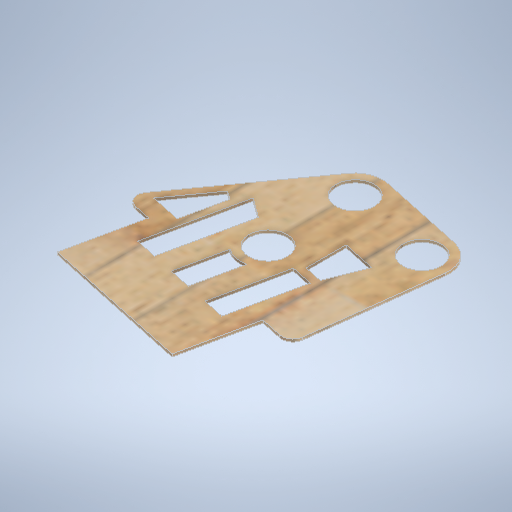
# Autodesk Inventor part: gear_plate_base
Saved by Autodesk Inventor 2026.1 (Build 301233020, 233B)
## iProperties
Created: 2024-04-01
Part Number: gear_plate_base
Material: 木材 (カエデ材)
Document SubType Name: Modeling
Designer: hibik
Density: 0.67 g/cm^3
Appearance: ナチュラル カエデ材 - 光沢 濃い着色
Author: hibik
Autodesk Inventor part; units mm, degrees
ref_plane "YZ Plane" through (0, 0, 0) normal (1, 0, 0) x (0, 1, 0)
ref_plane "XZ Plane" through (0, 0, 0) normal (0, 1, 0) x (-1, 0, 0)
ref_plane "XY Plane" through (0, 0, 0) normal (0, 0, 1) x (1, 0, 0)
sketch "スケッチ1" plane through (0, 0, 0) normal (0, 1, 0) x (-1, 0, 0)
  line L0 (25, 0) -> (-25, 0)
  line L1 (-25, 0) -> (-25, -104.5)
  line L2 (-25, -104.5) -> (25, -104.5) construction
  line L3 (25, -104.5) -> (25, 0)
  circle A0 centre (0, 0) radius 25
  circle A1 centre (0, 0) radius 57 construction
  circle A2 centre (0, -79.5) radius 22.5 construction
  circle A3 centre (0, 0) radius 75 construction
  circle A4 centre (0, -79.5) radius 10.75
  circle A5 centre (0, 0) radius 10.75
  circle A6 centre (-77.7461, -62.8931) radius 25
  circle A7 centre (-77.7461, -62.8931) radius 10.75
  circle A8 centre (0, -79.5) radius 25
  line L4 (-5.2223, -103.9485) -> (-82.9684, -87.3415)
  line L5 (-72.5238, -38.4446) -> (5.2223, -55.0515)
  line L6 (-77.7461, -62.8931) -> (-82.9684, -87.3415)
  point P0 (25, -79.5)
  point P1 (-25, -48.5959)
  dimension "d0" = 114
  dimension "d1" = 45
  dimension "d2" = 150
  dimension "d4" = 21.5
  dimension "d5" = 50
  dimension "d25" = 79.5
  constraints: 14 end point, 9 centre point, 9 tangent, 8 coincident, 5 point on circle, 3 equal radius, 2 parallel, 2 perpendicular, 1 horizontal, 1 midpoint, 1 vertical alignment
  measures "d0" diameter of A1
  measures "d1" diameter of A2
  measures "d2" diameter of A3
  measures "d4" diameter of A5
  measures "d5" distance of L1.end L2.end
  measures "d25" distance from line of A2.centre L6
extrude "押し出し1" add sketch "スケッチ1" along normal blind 2.5 contours A0 L0 A5 | L0 A5 A0 | L3 A8 L5 L1 A0 | A8 | A8 L1 L5 | L4 L1 A8 | L1 L4 A6 L5 | A6
sketch "スケッチ4" plane through (0, 2.5, 0) normal (0, 1, 0) x (1, 0, 0)
  line L0 (-1, 90.2034) -> (1, 90.2034)
  line L1 (1, 90.2034) -> (1, 96.5)
  line L2 (1, 96.5) -> (-1, 96.5)
  line L3 (-1, 96.5) -> (-1, 90.2034)
  arc A0 (-25, 0) -> (25, 0) centre (0, 0) ccw projected
  line L4 (25, 0) -> (25, 48.5959) projected
  line L5 (25, 48.5959) -> (72.5238, 38.4446) projected
  arc A1 (72.5238, 38.4446) -> (82.9684, 87.3415) centre (77.7461, 62.8931) ccw projected
  line L6 (82.9684, 87.3415) -> (5.2223, 103.9485) projected
  arc A2 (5.2223, 103.9485) -> (-25, 79.5) centre (0, 79.5) ccw projected
  line L7 (-25, 79.5) -> (-25, 0) projected
  circle A3 centre (0, 0) radius 10.75 projected
  circle A4 centre (77.7461, 62.8931) radius 10.75 projected
  circle A5 centre (0, 79.5) radius 10.75 projected
  circle A6 centre (0, 79.5) radius 10.75 projected
  line L8 (-16.9706, -1) -> (16.9706, -1)
  line L9 (16.9706, -1) -> (16.9706, 1)
  line L10 (16.9706, 1) -> (-16.9706, 1)
  line L11 (-16.9706, 1) -> (-16.9706, -1)
  line L12 (-1, -16.9706) -> (1, -16.9706)
  line L13 (1, -16.9706) -> (1, 16.9706)
  line L14 (1, 16.9706) -> (-1, 16.9706)
  line L15 (-1, 16.9706) -> (-1, -16.9706)
  circle A7 centre (0, 0) radius 17
  point P0 (0, 96.5)
  point P1 (-16.9706, 0)
  point P2 (0, 16.9706)
  point P3 (-1, -10.7034)
  point P4 (1, -10.7034)
  point P5 (10.7034, 1)
  point P6 (10.7034, -1)
  point P7 (-1, 10.7034)
  point P8 (1, 10.7034)
  point P9 (-10.7034, -1)
  point P10 (-10.7034, 1)
  dimension "d26" = 17
  dimension "d27" = 2
  dimension "d30" = 34
  constraints: 24 end point, 6 parallel, 5 perpendicular, 4 point on circle, 3 horizontal, 3 midpoint, 2 vertical alignment, 1 centre point, 1 coincident, 1 horizontal alignment, 2 other
  measures "d26" distance from line of L2 A2.centre
  measures "d27" distance of L1.end L2.end
  measures "d30" diameter of A7
extrude "押し出し4" cut sketch "スケッチ4" against normal through all contours A5 L0 | L3 L2 L1 A5 | A3 L10 L9 L8 | A3 L15 L14 L13 | L13 L12 L15 A3 | A3 L8 L11 L10 picked at (-0.1113, 90.2172)
sketch "スケッチ5" plane through (0, 2.5, 0) normal (0, 1, 0) x (1, 0, 0)
  circle A0 centre (0, 0) radius 17.5
  circle A1 centre (0, 79.5) radius 17.5
  circle A2 centre (77.7461, 62.8931) radius 17.5
  arc A3 (-1, 90.2034) -> (1, 90.2034) centre (0, 79.5) ccw projected
  circle A4 centre (77.7461, 62.8931) radius 10.75 projected
  dimension "d31" = 35
  dimension "d32" = 35
  dimension "d33" = 35
  constraints: 3 centre point, 2 concentric, 1 coincident
  measures "d31" diameter of A0
  measures "d32" diameter of A1
  measures "d33" diameter of A2
extrude "押し出し5" cut sketch "スケッチ5" against normal through all contours A0 | A1 | A2 | A4
sketch "スケッチ7" plane through (0, 2.5, 0) normal (0, 1, 0) x (1, 0, 0)
  line L0 (62.2228, 90.7503) -> (63.2008, 90.5415) projected
  line L1 (62.7118, 90.6459) -> (67.0985, 111.1826)
  line L2 (9.4001, 123.5072) -> (87.1463, 106.9003) projected
  circle A0 centre (50.445, 105.0256) radius 1.75
  circle A1 centre (21.1068, 111.2923) radius 1.75
  point P0 (0, 0)
  dimension "d39" = 9.5
  dimension "d40" = 3.5
  dimension "d41" = 15
  dimension "d42" = 45
  dimension "d43" = 9.5
  constraints: 2 centre point, 2 end point, 1 equal radius, 1 midpoint, 1 perpendicular, 1 point on line
  measures "d39" distance from line of A0.centre L2
  measures "d40" diameter of A0
  measures "d41" distance from line of L1 A0.centre
  measures "d42" distance from line of A1.centre L1
  measures "d43" distance from line of L2 A1.centre
extrude "押し出し7" cut sketch "スケッチ7" against normal through all
sketch "スケッチ8" plane through (0, 2.5, 0) normal (0, 1, 0) x (1, 0, 0)
  line L0 (15.7233, -19.4365) -> (93.4694, 43.4566)
  arc A0 (-25, 0) -> (25, 0) centre (0, 0) ccw projected
  arc A1 (72.5238, 38.4446) -> (82.9684, 87.3415) centre (77.7461, 62.8931) ccw projected
  line L1 (25, 0) -> (25, 42.4151) projected
  line L2 (25, 0) -> (25, 48.5959) projected
  line L3 (25, 48.5959) -> (72.5238, 38.4446) projected
  constraints: 2 end point, 2 point on circle, 2 tangent
extrude "押し出し8" add sketch "スケッチ8" against normal up to surface (2.5 mm away)
sketch "スケッチ11" plane through (0, 2.5, 0) normal (0, 1, 0) x (1, 0, 0)
  line L0 (57.451, -61.3546) -> (47.0063, -110.2515) projected
  line L1 (86.7891, -67.6214) -> (57.451, -61.3546) projected
  line L2 (57.5442, -204.5328) -> (86.7891, -67.6214) projected
  line L3 (42.8751, -201.3994) -> (57.5442, -204.5328) projected
  line L4 (58.542, -128.054) -> (42.8751, -201.3994) projected
  arc A0 (58.542, -128.054) -> (47.0063, -110.2515) centre (43.873, -124.9206) ccw projected
  arc A1 (-87.9492, -81.4244) -> (-105.7517, -92.9601) centre (-91.0826, -96.0935) ccw projected
  line L5 (-105.7517, -92.9601) -> (-121.4186, -166.3055) projected
  line L6 (-121.4186, -166.3055) -> (-136.0876, -163.1722) projected
  line L7 (-136.0876, -163.1722) -> (-106.8428, -26.2607) projected
  line L8 (-106.8428, -26.2607) -> (-77.5046, -32.5275) projected
  line L9 (-77.5046, -32.5275) -> (-87.9492, -81.4244) projected
  line L10 (-117.2874, -75.1577) -> (76.3445, -116.5183) projected
  line L11 (-111.0206, -45.8195) -> (-117.2874, -75.1577) projected
  line L12 (-81.6824, -52.0863) -> (-111.0206, -45.8195) projected
  line L13 (-84.8158, -66.7554) -> (-81.6824, -52.0863) projected
  line L14 (50.1397, -95.5825) -> (-84.8158, -66.7554) projected
  line L15 (53.2731, -80.9134) -> (50.1397, -95.5825) projected
  line L16 (82.6113, -87.1801) -> (53.2731, -80.9134) projected
  line L17 (76.3445, -116.5183) -> (82.6113, -87.1801) projected
  line L18 (-99.6213, -36.495) -> (-103.0441, -35.7639) projected
  line L19 (-103.0441, -35.7639) -> (-103.6708, -38.6977) projected
  line L20 (-103.6708, -38.6977) -> (-100.248, -39.4288) projected
  line L21 (-100.248, -39.4288) -> (-100.9791, -42.8516) projected
  line L22 (-100.9791, -42.8516) -> (-98.0453, -43.4783) projected
  line L23 (-98.0453, -43.4783) -> (-97.3142, -40.0555) projected
  line L24 (-97.3142, -40.0555) -> (-93.8914, -40.7866) projected
  line L25 (-93.8914, -40.7866) -> (-93.2647, -37.8528) projected
  line L26 (-93.2647, -37.8528) -> (-96.6875, -37.1217) projected
  line L27 (-96.6875, -37.1217) -> (-95.9564, -33.6989) projected
  line L28 (-95.9564, -33.6989) -> (-98.8902, -33.0722) projected
  line L29 (-98.8902, -33.0722) -> (-99.6213, -36.495) projected
  line L30 (69.0332, -75.5881) -> (72.456, -76.3192) projected
  line L31 (72.456, -76.3192) -> (71.7249, -79.742) projected
  line L32 (71.7249, -79.742) -> (74.6587, -80.3686) projected
  line L33 (74.6587, -80.3686) -> (75.3898, -76.9459) projected
  line L34 (75.3898, -76.9459) -> (78.8126, -77.677) projected
  line L35 (78.8126, -77.677) -> (79.4393, -74.7432) projected
  line L36 (79.4393, -74.7432) -> (76.0165, -74.012) projected
  line L37 (76.0165, -74.012) -> (76.7476, -70.5893) projected
  line L38 (76.7476, -70.5893) -> (73.8138, -69.9626) projected
  line L39 (73.8138, -69.9626) -> (73.0827, -73.3854) projected
  line L40 (73.0827, -73.3854) -> (69.6599, -72.6542) projected
  line L41 (69.6599, -72.6542) -> (69.0332, -75.5881) projected
  line L42 (-106.8428, -26.2607) -> (-111.0206, -45.8195) projected
  line L43 (86.7891, -67.6214) -> (-106.8428, -26.2607) projected
  line L44 (82.6113, -87.1801) -> (86.7891, -67.6214) projected
  line L45 (-111.0206, -45.8195) -> (82.6113, -87.1801) projected
  line L46 (86.7891, -67.6214) -> (102.557, 59.8234)
  arc A2 (93.4694, 43.4566) -> (82.9684, 87.3415) centre (77.7461, 62.8931) ccw projected
  line L47 (-106.8428, -26.2607) -> (-20.2972, 94.0953)
  arc A3 (5.2223, 103.9485) -> (-25, 79.5) centre (0, 79.5) ccw projected
  line L48 (-87.9492, -81.4244) -> (47.0063, -110.2515)
  line L49 (47.0063, -110.2515) -> (42.8285, -129.8103)
  line L50 (42.8285, -129.8103) -> (-92.127, -100.9832)
  line L51 (-92.127, -100.9832) -> (-87.9492, -81.4244)
  circle A4 centre (0, 0) radius 17.5 projected
  circle A5 centre (0, 79.5) radius 17.5 projected
  circle A6 centre (77.7461, 62.8931) radius 17.5 projected
  arc A7 (-25, 0) -> (15.7233, -19.4365) centre (0, 0) ccw projected
  line L52 (-25, 79.5) -> (-25, 0) projected
  arc A8 (5.2223, 103.9485) -> (-25, 79.5) centre (0, 79.5) ccw projected
  line L53 (82.9684, 87.3415) -> (5.2223, 103.9485) projected
  arc A9 (93.4694, 43.4566) -> (82.9684, 87.3415) centre (77.7461, 62.8931) ccw projected
  line L54 (93.4694, 43.4566) -> (15.7233, -19.4365) projected
  point P0 (-25, 79.5)
  dimension "d60" = 20
  constraints: 12 end point, 2 parallel, 2 perpendicular, 2 point on circle, 2 tangent
  measures "d60" distance between parallel lines of L50 L10
extrude "押し出し11" add sketch "スケッチ11" against normal up to surface (2.5 mm away) contours L43 L8 L47 A3 L52 A7 L54 A2 L46 L1 | L0 L45 L9 L43 | L0 L14 L9 L45 | L0 L10 L9 L14 | L49 L50 L51 L10
sketch "スケッチ12" plane through (0, 2.5, 0) normal (0, 1, 0) x (1, 0, 0)
  circle A0 centre (0, 0) radius 17.5 projected
  circle A1 centre (0, 79.5) radius 17.5 projected
  circle A2 centre (77.7461, 62.8931) radius 17.5 projected
  line L0 (-20.2972, 94.0953) -> (-106.8428, -26.2607) projected
  line L1 (-106.8428, -26.2607) -> (-77.5046, -32.5275) projected
  line L2 (-77.5046, -32.5275) -> (-92.127, -100.9832) projected
  line L3 (-92.127, -100.9832) -> (42.8285, -129.8103) projected
  line L4 (42.8285, -129.8103) -> (57.451, -61.3546) projected
  line L5 (57.451, -61.3546) -> (86.7891, -67.6214) projected
  line L6 (86.7891, -67.6214) -> (102.557, 59.8234) projected
  arc A3 (102.557, 59.8234) -> (82.9684, 87.3415) centre (77.7461, 62.8931) ccw projected
  line L7 (82.9684, 87.3415) -> (5.2223, 103.9485) projected
  arc A4 (5.2223, 103.9485) -> (-20.2972, 94.0953) centre (0, 79.5) ccw projected
  line L8 (-91.1491, -101.1921) -> (-76.5267, -32.7364)
  line L9 (-76.5267, -32.7364) -> (56.473, -61.1457)
  line L10 (56.473, -61.1457) -> (41.8506, -129.6014)
  line L11 (41.8506, -129.6014) -> (-91.1491, -101.1921)
  line L12 (-92.127, -100.9832) -> (42.8285, -129.8103) projected
  line L13 (-76.5267, -32.7364) -> (-77.5046, -32.5275)
  line L14 (56.473, -61.1457) -> (57.451, -61.3546)
  point P0 (-43.3372, -30.9427)
  dimension "d63" = 1
  dimension "d64" = 1
  constraints: 12 end point, 3 point on line, 2 parallel, 1 collinear, 1 perpendicular, 1 other
  measures "d63" distance between parallel lines of L2 L8
  measures "d64" distance between parallel lines of L4 L10
extrude "押し出し12" cut sketch "スケッチ12" against normal through all contours A0 | L13 L8 L3 L2 | L14 L4 L3 L10
sketch "スケッチ13" plane through (0, 2.5, 0) normal (0, 1, 0) x (1, 0, 0)
  arc A0 (-25, 0) -> (25, 0) centre (0, 0) ccw projected
  line L0 (25, 0) -> (25, 42.4151) projected
  arc A1 (31.0445, 47.3048) -> (25, 42.4151) centre (30, 42.4151) ccw projected
  line L1 (31.0445, 47.3048) -> (72.5238, 38.4446) projected
  arc A2 (72.5238, 38.4446) -> (82.9684, 87.3415) centre (77.7461, 62.8931) ccw projected
  line L2 (82.9684, 87.3415) -> (5.2223, 103.9485) projected
  arc A3 (5.2223, 103.9485) -> (-25, 79.5) centre (0, 79.5) ccw projected
  line L3 (-25, 79.5) -> (-25, 0) projected
  line L4 (-1, 90.2034) -> (-1, 96.5) projected
  line L5 (-1, 96.5) -> (1, 96.5) projected
  line L6 (1, 96.5) -> (1, 90.2034) projected
  arc A4 (10.7034, 80.5) -> (1, 90.2034) centre (0, 79.5) ccw projected
  line L7 (10.7034, 80.5) -> (16.9706, 80.5) projected
  line L8 (16.9706, 80.5) -> (16.9706, 78.5) projected
  line L9 (16.9706, 78.5) -> (10.7034, 78.5) projected
  arc A5 (-10.7034, 78.5) -> (10.7034, 78.5) centre (0, 79.5) ccw projected
  line L10 (-10.7034, 78.5) -> (-16.9706, 78.5) projected
  line L11 (-16.9706, 78.5) -> (-16.9706, 80.5) projected
  line L12 (-16.9706, 80.5) -> (-10.7034, 80.5) projected
  arc A6 (-1, 90.2034) -> (-10.7034, 80.5) centre (0, 79.5) ccw projected
  line L13 (60.7756, 63.8931) -> (67.0427, 63.8931) projected
  arc A7 (76.7461, 73.5965) -> (67.0427, 63.8931) centre (77.7461, 62.8931) ccw projected
  line L14 (76.7461, 73.5965) -> (76.7461, 79.8636) projected
  line L15 (76.7461, 79.8636) -> (78.7461, 79.8636) projected
  line L16 (78.7461, 79.8636) -> (78.7461, 73.5965) projected
  arc A8 (88.4495, 63.8931) -> (78.7461, 73.5965) centre (77.7461, 62.8931) ccw projected
  line L17 (88.4495, 63.8931) -> (94.7167, 63.8931) projected
  line L18 (94.7167, 63.8931) -> (94.7167, 61.8931) projected
  line L19 (94.7167, 61.8931) -> (88.4495, 61.8931) projected
  arc A9 (78.7461, 52.1897) -> (88.4495, 61.8931) centre (77.7461, 62.8931) ccw projected
  line L20 (78.7461, 52.1897) -> (78.7461, 45.9225) projected
  line L21 (78.7461, 45.9225) -> (76.7461, 45.9225) projected
  line L22 (76.7461, 45.9225) -> (76.7461, 52.1897) projected
  arc A10 (67.0427, 61.8931) -> (76.7461, 52.1897) centre (77.7461, 62.8931) ccw projected
  line L23 (67.0427, 61.8931) -> (60.7756, 61.8931) projected
  line L24 (60.7756, 61.8931) -> (60.7756, 63.8931) projected
  line L25 (-16.9706, 1) -> (-10.7034, 1) projected
  arc A11 (-1, 10.7034) -> (-10.7034, 1) centre (0, 0) ccw projected
  line L26 (-1, 10.7034) -> (-1, 16.9706) projected
  line L27 (-1, 16.9706) -> (1, 16.9706) projected
  line L28 (1, 16.9706) -> (1, 10.7034) projected
  arc A12 (10.7034, 1) -> (1, 10.7034) centre (0, 0) ccw projected
  line L29 (10.7034, 1) -> (16.9706, 1) projected
  line L30 (16.9706, 1) -> (16.9706, -1) projected
  line L31 (16.9706, -1) -> (10.7034, -1) projected
  arc A13 (1, -10.7034) -> (10.7034, -1) centre (0, 0) ccw projected
  line L32 (1, -10.7034) -> (1, -16.9706) projected
  line L33 (1, -16.9706) -> (-1, -16.9706) projected
  line L34 (-1, -16.9706) -> (-1, -10.7034) projected
  arc A14 (-10.7034, -1) -> (-1, -10.7034) centre (0, 0) ccw projected
  line L35 (-10.7034, -1) -> (-16.9706, -1) projected
  line L36 (-16.9706, -1) -> (-16.9706, 1) projected
  point P0 (0, 0)
sketch "スケッチ14" plane through (0, 2.5, 0) normal (0, 1, 0) x (1, 0, 0)
  line L0 (-84.4832, -41.2624) -> (-86.5721, -51.0418) construction
  line L1 (-86.5721, -51.0418) -> (58.1628, -81.9578) construction
  line L2 (58.1628, -81.9578) -> (60.2517, -72.1785) construction
  line L3 (60.2517, -72.1785) -> (-84.4832, -41.2624) construction
  line L4 (50.1397, -95.5825) -> (-84.8158, -66.7554) construction
  line L5 (-83.8379, -66.9643) -> (-80.7045, -52.2952)
  line L6 (-80.7045, -52.2952) -> (52.2952, -80.7045)
  line L7 (52.2952, -80.7045) -> (49.1618, -95.3736)
  line L8 (49.1618, -95.3736) -> (-83.8379, -66.9643)
  line L9 (-76.5267, -32.7364) -> (-91.1491, -101.1921) projected
  line L10 (41.8506, -129.6014) -> (56.473, -61.1457) projected
  line L11 (-63.1016, -56.0552) -> (-43.5428, -60.2331)
  line L12 (-43.5428, -60.2331) -> (-25, 26.5761)
  line L13 (-25, 26.5761) -> (-44.5588, 30.7539)
  line L14 (-44.5588, 30.7539) -> (-63.1016, -56.0552)
  line L15 (-23.984, -64.4109) -> (-4.4253, -68.5888)
  line L16 (-4.4253, -68.5888) -> (9.7794, -2.0889)
  line L17 (9.7794, -2.0889) -> (-9.7794, 2.0889)
  line L18 (-9.7794, 2.0889) -> (-23.984, -64.4109)
  line L19 (15.1335, -72.7666) -> (34.6923, -76.9444)
  line L20 (34.6923, -76.9444) -> (48.8969, -10.4446)
  line L21 (48.8969, -10.4446) -> (29.3382, -6.2668)
  line L22 (29.3382, -6.2668) -> (15.1335, -72.7666)
  line L23 (-25, 79.5) -> (-25, 0) projected
  arc A0 (-25, 0) -> (25, 0) centre (0, 0) ccw projected
  line L24 (25, 0) -> (25, 42.4151) projected
  arc A1 (31.0445, 47.3048) -> (25, 42.4151) centre (30, 42.4151) ccw projected
  line L25 (31.0445, 47.3048) -> (72.5238, 38.4446) projected
  arc A2 (72.5238, 38.4446) -> (82.9684, 87.3415) centre (77.7461, 62.8931) ccw projected
  arc A3 (5.2223, 103.9485) -> (-25, 79.5) centre (0, 79.5) ccw projected
  line L26 (-44.5588, 30.7539) -> (-58.5897, 40.8432)
  line L27 (-20.2972, 94.0953) -> (-106.8428, -26.2607) projected
  line L28 (-44.5588, 30.7539) -> (-25, 16.6896)
  line L29 (-63.2874, 25.7459) -> (-54.1846, 19.2002)
  line L30 (-54.1846, 19.2002) -> (-62.6359, -20.3651)
  line L31 (-62.6359, -20.3651) -> (-89.8079, -14.5611)
  line L32 (-89.8079, -14.5611) -> (-61.6636, 24.5782)
  line L33 (-106.8428, -26.2607) -> (-76.5267, -32.7364) projected
  line L34 (35, -0.3182) -> (35, 36.2343)
  line L35 (64.7587, 29.8777) -> (51.4944, -3.8415)
  line L36 (51.4944, -3.8415) -> (35, -0.3182)
  line L37 (85.8337, -18.3345) -> (81.7662, -51.2101)
  line L38 (48.8491, -44.1788) -> (55.7425, -11.9068)
  line L39 (35, 36.2343) -> (64.7587, 29.8777)
  line L40 (86.7891, -67.6214) -> (102.557, 59.8234) projected
  line L41 (81.7662, -51.2101) -> (48.8491, -44.1788)
  line L42 (86.7891, -67.6214) -> (56.473, -61.1457) projected
  line L43 (55.7425, -11.9068) -> (85.8337, -18.3345)
  line L44 (58.4335, -5.3237) -> (72.4996, 30.4337)
  line L45 (72.4996, 30.4337) -> (92.0411, 31.8375)
  line L46 (92.0411, 31.8375) -> (86.6965, -11.3608)
  line L47 (86.6965, -11.3608) -> (58.4335, -5.3237)
  point P0 (0, 0)
  point P1 (-83.8379, -66.9643)
  point P2 (-14.2047, -66.4998)
  point P3 (0, 0)
  point P4 (4.9931, -24.4963)
  point P5 (-14.5657, -20.3185)
  point P6 (-26.8306, 18.006)
  dimension "d68" = 20
  dimension "d69" = 20
  dimension "d70" = 20
  dimension "d75" = 7
  dimension "d76" = 15
  dimension "d77" = 7
  dimension "d78" = 15
  dimension "d79" = 7
  dimension "d80" = 10
  dimension "d81" = 10
  dimension "d82" = 7
  dimension "d83" = 7
  dimension "d84" = 15
  dimension "d85" = 7
  dimension "d86" = 7
  dimension "d87" = 7
  dimension "d88" = 32
  constraints: 68 end point, 21 parallel, 17 point on line, 7 perpendicular, 6 midpoint, 2 collinear, 2 equal length
  measures "d68" distance between parallel lines of L16 L18
  measures "d69" distance between parallel lines of L12 L18
  measures "d70" distance between parallel lines of L22 L16
  measures "d75" distance between parallel lines of L27 L32
  measures "d76" distance between parallel lines of L26 L29
  measures "d77" distance between parallel lines of L14 L30
  measures "d78" distance between parallel lines of L33 L31
  measures "d79" distance between parallel lines of L36 L21
  measures "d80" distance between parallel lines of L24 L34
  measures "d81" distance between parallel lines of L25 L39
  measures "d82" distance between parallel lines of L20 L38
  measures "d83" distance between parallel lines of L40 L37
  measures "d84" distance between parallel lines of L42 L41
  measures "d85" distance between parallel lines of L35 L44
  measures "d86" distance between parallel lines of L43 L47
  measures "d87" distance between parallel lines of L40 L46
  measures "d88" distance from line of A2.centre L45
fillet "フィレット1" radius 10 2 edges at (86.7891, 1.25, 67.6214) (-106.8428, 1.25, 26.2607)
extrude "押し出し13" cut sketch "スケッチ14" against normal through all contours L14 L28 L12 L6 | L6 L22 L21 L20 | L18 A0 L16 L6 | L29 L30 L31 L32 | L34 L39 L35 L36
equation "\"d43\" = d39"
equation "\"d64\" = d63"
equation "\"d70\" = d69"
equation "\"d77\" = d75"
equation "\"d78\" = d76"
equation "\"d79\" = d75"
equation "\"d80\" = d81"
equation "\"d82\" = d77"
equation "\"d83\" = d75"
equation "\"d84\" = d78"
equation "\"d85\" = d83"
equation "\"d86\" = d83"
equation "\"d87\" = d83"
